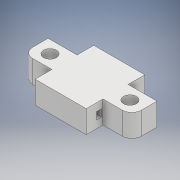
# Autodesk Inventor part: Finger juncture
Saved by Autodesk Inventor 2018 (Build 220112000, 112)
## iProperties
Created: 2018-02-19
Part Number: Finger juncture
Material: Plastique ABS
Document SubType Name: Modeling
Designer: Thomas
Density: 1.06 g/cm^3
Appearance: Lisse - Blanc
Author: Thomas
Autodesk Inventor part; units mm, degrees
ref_plane "YZ Plane" through (0, 0, 0) normal (1, 0, 0) x (0, 1, 0)
ref_plane "XZ Plane" through (0, 0, 0) normal (0, 1, 0) x (-1, 0, 0)
ref_plane "XY Plane" through (0, 0, 0) normal (0, 0, 1) x (1, 0, 0)
sketch "Esquisse1" plane through (0, 0, 0) normal (0, 0, 1) x (1, 0, 0)
  line L0 (0, 0) -> (0, 7.8)
  line L1 (0, 7.8) -> (8.97, 7.8)
  line L2 (8.97, 7.8) -> (8.97, 13)
  line L3 (8.97, 13) -> (24.83, 13)
  line L4 (24.83, 13) -> (24.83, 7.8)
  line L5 (24.83, 7.8) -> (33.8, 7.8)
  line L6 (33.8, 7.8) -> (33.8, 0)
  line L7 (33.8, 0) -> (24.83, 0)
  line L8 (24.83, 0) -> (24.83, -5.2)
  line L9 (24.83, -5.2) -> (8.97, -5.2)
  line L10 (8.97, -5.2) -> (8.97, 0)
  line L11 (0, 0) -> (8.97, 0)
  dimension "d0" = 7.8
  dimension "d1" = 7.8
  dimension "d2" = 15.86
  dimension "d3" = 33.8
  dimension "d4" = 18.2
  dimension "d5" = 5.2
  dimension "d6" = 8.97
  constraints: 24 end point, 7 perpendicular, 7 point on line, 1 vertical
  measures "d0" distance of L0.start L0.end
  measures "d1" distance of L5.end L6.end
  measures "d2" distance of L2.end L3.end
  measures "d3" distance between parallel lines of L6 L0
  measures "d4" distance between parallel lines of L9 L3
  measures "d5" distance between parallel lines of L3 L1
  measures "d6" distance between parallel lines of L2 L0
extrude "Extrusion1" add sketch "Esquisse1" along normal blind 7
sketch "Esquisse2" plane through (0, 0, 7) normal (0, 0, 1) x (1, 0, 0)
  line L0 (0, 7.8) -> (0, 0) construction
  line L1 (0, 0) -> (8.97, 0) construction
  line L2 (0, 7.8) -> (8.97, 0) construction
  line L3 (8.97, 13) -> (8.97, 7.8) construction
  line L4 (8.97, 7.8) -> (0, 0) construction
  line L5 (24.83, 7.8) -> (33.8, 0) construction
  line L6 (33.8, 0) -> (33.8, 7.8) construction
  line L7 (24.83, -5.2) -> (24.83, 0) construction
  line L8 (33.8, 7.8) -> (24.83, 0) construction
  circle A0 centre (4.485, 3.9) radius 2
  circle A1 centre (29.315, 3.9) radius 2
  dimension "d9" = 4
  dimension "d10" = 4
  constraints: 8 end point, 2 centre point, 2 midpoint
  measures "d9" diameter of A0
  measures "d10" diameter of A1
extrude "Extrusion2" cut sketch "Esquisse2" against normal blind 7
fillet "Congé1" radius 3 1 edges at (0, 0, 3.5)
fillet "Congé2" radius 3 1 edges at (33.8, 0, 3.5)
sketch "Esquisse3" plane through (24.83, 7.8, 0) normal (1, 0, 0) x (0, 0, -1)
  line L0 (-4.6, 2) -> (-2.4, 2)
  line L1 (-2.4, 2) -> (-2.4, 0.5)
  line L2 (-2.4, 0.5) -> (-4.6, 0.5)
  line L3 (-4.6, 0.5) -> (-4.6, 2)
  line L4 (-4.6, -8.3) -> (-2.4, -8.3)
  line L5 (-2.4, -8.3) -> (-2.4, -9.8)
  line L6 (-2.4, -9.8) -> (-4.6, -9.8)
  line L7 (-4.6, -9.8) -> (-4.6, -8.3)
  line L8 (0, -7.8) -> (-7, -7.8) projected
  line L9 (0, -7.8) -> (0, -13) projected
  line L10 (0, 0) -> (-7, 0) projected
  dimension "d15" = 2.2
  dimension "d16" = 1.5
  dimension "d17" = 0.5
  dimension "d18" = 2.4
  dimension "d19" = 0.5
  dimension "d20" = 1.5
  constraints: 16 end point, 4 parallel, 2 horizontal, 2 perpendicular, 2 point on line
  measures "d15" distance of L5.end L6.end
  measures "d16" distance of L4.end L5.end
  measures "d17" distance between parallel lines of L8 L4
  measures "d18" distance between parallel lines of L9 L5
  measures "d19" distance between parallel lines of L2 L10
  measures "d20" distance of L0.end L1.end
extrude "Extrusion3" cut sketch "Esquisse3" against normal blind 15.86
